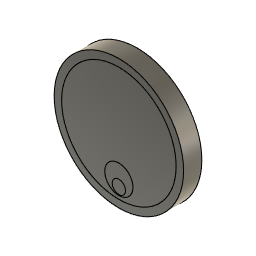
Plato v3 (Autodesk Fusion 360 design; units mm, degrees)
Autodesk Fusion 360 part; units mm, degrees
sketch "Sketch2" plane through (0, 0, 0) normal (0, 1, 0) x (1, 0, 0)
  circle A0 centre (0, 0) radius 195
  circle A1 centre (0, 0) radius 172.5
  circle A2 centre (0, 120) radius 42.4264
  circle A3 centre (0, 140) radius 20
  dimension "d11" = 390
  dimension "d12" = 345
  constraint coincident A0.centre A1.centre
  constraint concentric A0 A1
  measures "d11" diameter of A0
  measures "d12" diameter of A1
extrude "Extrude5" add sketch "Sketch2" along normal blind 55 contours A0 makes body 1
extrude "Extrude6" add sketch "Sketch2" along normal blind 55 separate body contours A1 makes body 2
extrude "Extrude7" add sketch "Sketch2" along normal blind 55 separate body contours A2 makes body 3
extrude "Extrude8" add sketch "Sketch2" along normal blind 54 separate body contours A3 makes body 4
